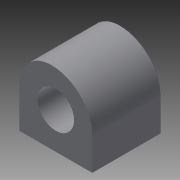
# Autodesk Inventor part: Gounded Clevis
Saved by Autodesk Inventor 2015 (Build 190159000, 159)
## iProperties
Created: 2016-01-11
Part Number: Gounded Clevis
Material: Generic
Document SubType Name: Modeling
Designer: Applegate
Density: 1 g/cm^3
Appearance: Default
Author: Applegate
Autodesk Inventor part; units mm, degrees
ref_plane "YZ Plane" through (0, 0, 0) normal (1, 0, 0) x (0, 1, 0)
ref_plane "XZ Plane" through (0, 0, 0) normal (0, 1, 0) x (-1, 0, 0)
ref_plane "XY Plane" through (0, 0, 0) normal (0, 0, 1) x (1, 0, 0)
sketch "Sketch1" plane through (0, 0, 0) normal (0, 1, 0) x (-1, 0, 0)
  line L0 (-12.7, 11.9062) -> (12.7, 11.9062)
  line L1 (12.7, 11.9062) -> (12.7, -11.9062)
  line L2 (12.7, -11.9062) -> (-12.7, -11.9062)
  line L3 (-12.7, -11.9062) -> (-12.7, 11.9062)
  point P0 (0, 0)
  point P1 (-12.7, 0)
  point P2 (0, 11.9062)
  dimension "d0" = 25.4
  dimension "d1" = 23.8125
  constraints: 8 end point, 2 midpoint, 2 parallel, 1 horizontal, 1 horizontal alignment, 1 perpendicular, 1 vertical alignment
  measures "d0" distance of L1.end L2.end
  measures "d1" distance of L0.end L1.end
extrude "Extrusion1" add sketch "Sketch1" along normal blind 25.4
sketch "Sketch2" plane through (-12.7, 0, 11.9062) normal (0, 0, 1) x (1, 0, 0)
  circle A0 centre (12.7, 12.7) radius 6.35
  line L0 (0, 0) -> (0, 25.4) projected
  line L1 (25.4, 0) -> (0, 0) projected
  point P0 (12.7, 0)
  point P1 (0, 12.7)
  point P2 (12.7, 0)
  dimension "d4" = 12.7
  constraints: 2 midpoint, 1 centre point, 1 horizontal alignment, 1 vertical alignment
  measures "d4" diameter of A0
extrude "Extrusion2" cut sketch "Sketch2" against normal blind 50.8
fillet "Fillet1" radius 14.2875 1 edges at (12.7, 25.4, 0)
fillet "Fillet2" radius 11.1125 1 edges at (-12.7, 25.4, 0)
body "Solid1"
